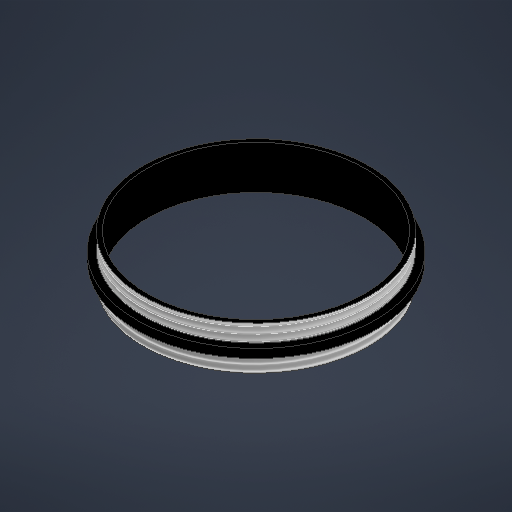
# Autodesk Inventor part: 77mm to 52mm
Saved by Autodesk Inventor 2026 (Build 300175000, 175)
## iProperties
Created: 2025-11-17
Part Number: 77mm to 52mm
Material: Aluminum 6061-AHC
Document SubType Name: Modeling
Designer: FiolkaLab
Mass: 41.9376 g
Surface Area: 101.568 cm^2
Volume: 15.5324 cm^3
Density: 2.7 g/cm^3
Appearance: Aluminum - Dark
Author: FiolkaLab
Autodesk Inventor part; units mm, degrees
ref_plane "YZ Plane" through (0, 0, 0) normal (1, 0, 0) x (0, 1, 0)
ref_plane "XZ Plane" through (0, 0, 0) normal (0, 1, 0) x (-1, 0, 0)
ref_plane "XY Plane" through (0, 0, 0) normal (0, 0, 1) x (1, 0, 0)
sketch "Sketch5" plane through (0, 0, 0) normal (0, 1, 0) x (-1, 0, 0)
  circle A0 centre (0, 0) radius 27.5
  dimension "d18" = 55
  constraints: 1 centre point, 1 coincident
  measures "d18" diameter of A0
extrude "Extrusion5" add sketch "Sketch5" along normal blind 2
sketch "Sketch6" plane through (0, 2, 0) normal (0, 1, 0) x (1, 0, 0)
  circle A0 centre (0, 0) radius 26
  dimension "d21" = 52
  constraints: 1 centre point, 1 coincident
  measures "d21" diameter of A0
extrude "Extrusion6" add sketch "Sketch6" along normal blind 4
sketch "Sketch7" plane through (0, 6, 0) normal (0, 1, 0) x (1, 0, 0)
  circle A0 centre (0, 0) radius 25
  dimension "d24" = 50
  constraints: 1 centre point, 1 coincident
  measures "d24" diameter of A0
extrude "Extrusion7" cut sketch "Sketch7" against normal through all
thread "Thread4" size "M52x1.5" class "6g" standard "ISO Metric profile" full length
sketch "Sketch8" plane through (0, 0, 0) normal (0, -1, 0) x (1, 0, 0)
  circle A0 centre (0, 0) radius 26
  dimension "d29" = 52
  constraints: 1 centre point, 1 coincident
  measures "d29" diameter of A0
extrude "Extrusion8" add sketch "Sketch8" along normal blind 4
sketch "Sketch9" plane through (0, -4, 0) normal (0, -1, 0) x (1, 0, 0)
  circle A0 centre (0, 0) radius 25
  dimension "d32" = 50
  constraints: 1 centre point, 1 coincident
  measures "d32" diameter of A0
extrude "Extrusion9" cut sketch "Sketch9" against normal blind 4
thread "Thread5" size "M52x1.5" class "6g" standard "ISO Metric profile" full length
body "Solid2"
